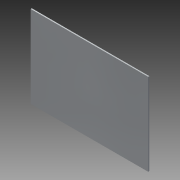
# Autodesk Inventor part: szyba
Saved by Autodesk Inventor 2013 (Build 170138000, 138)
## iProperties
Created: 2013-08-20
Part Number: szyba
Material: Szkło
Document SubType Name: Konstrukcja blachowa
Designer: Kisieel
Density: 1 g/cm^3
Flat Pattern Width: 0.3 cm
Flat Pattern Length: 21 cm
Flat Pattern Area: 6.3 cm^2
Sheet Metal Rule: Domyślny
Sheet Metal Width: 3,000 mm
Sheet Metal Length: 210,000 mm
Sheet Metal Area: 630,000 mm^2
Author: Kisieel
Autodesk Inventor part; units mm, degrees
ref_plane "YZ Plane" through (0, 0, 0) normal (1, 0, 0) x (0, 1, 0)
ref_plane "XZ Plane" through (0, 0, 0) normal (0, 1, 0) x (-1, 0, 0)
ref_plane "XY Plane" through (0, 0, 0) normal (0, 0, 1) x (1, 0, 0)
sketch "Szkic1" plane through (0, 0, 0) normal (0, 1, 0) x (-1, 0, 0)
  line L0 (-150, 105) -> (150, 105)
  line L1 (150, 105) -> (150, -105)
  line L2 (150, -105) -> (-150, -105)
  line L3 (-150, -105) -> (-150, 105)
  line L4 (0, -147) -> (0, 147) projected
  line L5 (210, 0) -> (-210, 0) projected
  point P0 (0, 0)
  dimension "d0" = 300
  dimension "d2" = 210
  constraints: 8 end point, 2 parallel, 1 horizontal, 1 perpendicular, 2 other
  measures "d0" distance of L0.start L0.end
  measures "d2" distance of L0.end L1.end
extrude "Wyciągnięcie proste1" add sketch "Szkic1" along normal blind 3
equation "\"PromieńGięcia\" = Grubość"
equation "\"SzerokośćGięciaPodcięcia\" = Grubość"
equation "\"GłębokośćGięciaPodcięcia\" = 0.5 * Grubość"
equation "\"RozmiarPodcięciaNarożnika\" = 4 * Grubość"
equation "\"MinimalnaPozostałość\" = 2 * Grubość"
equation "\"PromieńPrzejścia\" = PromieńGięcia"
equation "\"Rozmiar_promienia_Jacobiego\" = Grubość"
equation "\"Wielk_odstępu\" = Grubość"
equation "\"Grubość\" = 4"
